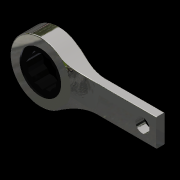
# Autodesk Inventor part: Ratchet
Saved by Autodesk Inventor 2014 SP1 (Build 180222100, 222)
## iProperties
Created: 2014-01-19
Part Number: Ratchet
Material: Generic
Document SubType Name: Modeling
Designer: Rauhul Varma
Mass: 5.86952 g
Surface Area: 33.2003 cm^2
Volume: 5.86952 cm^3
Density: 1 g/cm^3
Appearance: Steel - Polished
Author: Rauhul Varma
Autodesk Inventor part; units mm, degrees
ref_plane "YZ Plane" through (0, 0, 0) normal (1, 0, 0) x (0, 1, 0)
ref_plane "XZ Plane" through (0, 0, 0) normal (0, 1, 0) x (-1, 0, 0)
ref_plane "XY Plane" through (0, 0, 0) normal (0, 0, 1) x (1, 0, 0)
sketch "Sketch1" plane through (0, 0, 0) normal (0, 0, 1) x (1, 0, 0)
  arc A0 (12.3578, 6.35) -> (12.3578, -6.35) centre (0, 0) ccw
  line L0 (7.3323, 0) -> (3.6662, -6.35)
  line L1 (3.6662, -6.35) -> (-3.6662, -6.35)
  line L2 (-3.6662, -6.35) -> (-7.3323, 0)
  line L3 (-7.3323, 0) -> (-3.6662, 6.35)
  line L4 (-3.6662, 6.35) -> (3.6662, 6.35)
  line L5 (3.6662, 6.35) -> (7.3323, 0)
  line L6 (6.35, 3.6662) -> (6.35, -3.6662)
  line L7 (6.35, -3.6662) -> (0, -7.3323)
  line L8 (0, -7.3323) -> (-6.35, -3.6662)
  line L9 (-6.35, -3.6662) -> (-6.35, 3.6662)
  line L10 (-6.35, 3.6662) -> (0, 7.3323)
  line L11 (0, 7.3323) -> (6.35, 3.6662)
  line L12 (3.6662, 6.35) -> (12.3578, 6.35)
  line L13 (3.6662, -6.35) -> (12.3578, -6.35)
  line L14 (50.8, -6.35) -> (50.8, 6.35)
  line L15 (12.3578, 6.35) -> (50.8, 6.35)
  line L16 (12.3578, -6.35) -> (50.8, -6.35)
  arc A1 (12.3578, -6.35) -> (12.3578, 6.35) centre (0, 0) ccw
  dimension "d0" = 27.7876
  dimension "d1" = 12.7
  dimension "d2" = 12.7
  dimension "d14" = 50.8
  constraints: 34 end point, 4 parallel, 4 point on circle, 3 coincident, 2 centre point, 2 perpendicular, 2 vertical, 1 horizontal, 26 other
  measures "d0" diameter of A0
  measures "d1" distance between parallel lines of L1 L4
  measures "d2" distance between parallel lines of L8 L11
  measures "d14" distance from line of L14 A0.centre
extrude "Extrusion1" add sketch "Sketch1" along normal blind 4.3498 contours L12 L4 L11 L10 L3 L9 L2 L8 L1 L7 L13 A0 | A1 L13 L0 L7 L6 L5 L11 L12 | L5 L11 L4 | L1 L7 L0 | L11 L5 L6 L0 L7 L1 L8 L2 L9 L3 L10 L4 | L4 L10 L11 | L11 L6 L5 | L0 L6 L7 | L7 L8 L1 | L10 L3 L4 | L5 L0 L6 | L1 L2 L8 | L3 L9 L10 | L8 L9 L2 | L9 L2 L3
extrude "Extrusion2" add sketch "Sketch1" along normal blind 1.9685 contours A1 L13 L0 L7 L6 L5 L11 L12 | L15 L14 L16 A1 | L11 L6 L5 | L0 L6 L7
fillet "Fillet1" radius 25.4 3 edges at (12.3578, 6.35, 0.9842) (12.3578, -6.35, 0.9842) (13.8938, 0, 1.9685)
fillet "Fillet2" radius 0.3969 7 edges at (23.4746, 6.35, 1.9704) (15.2626, 7.6058, 3.1255) (37.2994, 6.35, 1.9685) (-13.8938, 0, 4.3498) (23.4746, -6.35, 1.9704) (37.2994, -6.35, 1.9685) (15.2626, -7.6058, 3.1255)
extrude "Extrusion3" cut sketch "Sketch1" along normal through all contours L5 L11 L4 | L1 L7 L0 | L11 L5 L6 L0 L7 L1 L8 L2 L9 L3 L10 L4 | L4 L10 L11 | L11 L6 L5 | L0 L6 L7 | L7 L8 L1 | L10 L3 L4 | L5 L0 L6 | L1 L2 L8 | L3 L9 L10 | L8 L9 L2 | L9 L2 L3
sketch "Sketch2" plane through (0, 0, 4.3498) normal (0, 0, 1) x (1, 0, 0)
  arc A0 (10.1891, -9.4457) -> (10.1891, 9.4457) centre (0, 0) ccw projected
  line L0 (6.35, 3.6662) -> (6.35, -3.6662) projected
  line L1 (6.35, -3.6662) -> (0, -7.3323) projected
  line L2 (4.6485, -4.6485) -> (3.6662, -6.35) projected
  line L3 (3.6662, -6.35) -> (1.7015, -6.35) projected
  line L4 (6.35, -3.6662) -> (0, -7.3323) projected
  line L5 (0, -7.3323) -> (-6.35, -3.6662) projected
  line L6 (-1.7015, -6.35) -> (-3.6662, -6.35) projected
  line L7 (-3.6662, -6.35) -> (-4.6485, -4.6485) projected
  line L8 (0, -7.3323) -> (-6.35, -3.6662) projected
  line L9 (-6.35, -3.6662) -> (-6.35, 3.6662) projected
  line L10 (-6.35, -1.7015) -> (-7.3323, 0) projected
  line L11 (-7.3323, 0) -> (-6.35, 1.7015) projected
  line L12 (-6.35, -3.6662) -> (-6.35, 3.6662) projected
  line L13 (-6.35, 3.6662) -> (0, 7.3323) projected
  line L14 (-4.6485, 4.6485) -> (-3.6662, 6.35) projected
  line L15 (-3.6662, 6.35) -> (-1.7015, 6.35) projected
  line L16 (-6.35, 3.6662) -> (0, 7.3323) projected
  line L17 (0, 7.3323) -> (6.35, 3.6662) projected
  line L18 (1.7015, 6.35) -> (3.6662, 6.35) projected
  line L19 (3.6662, 6.35) -> (4.6485, 4.6485) projected
  line L20 (0, 7.3323) -> (6.35, 3.6662) projected
  line L21 (6.35, 3.6662) -> (6.35, -3.6662) projected
  line L22 (6.35, 1.7015) -> (7.3323, 0) projected
  line L23 (7.3323, 0) -> (6.35, -1.7015) projected
  circle A1 centre (0, 0) radius 9.525
  dimension "d11" = 19.05
  constraints: 1 centre point, 1 coincident
  measures "d11" diameter of A1
extrude "Extrusion4" cut sketch "Sketch2" against normal blind 0.7937
sketch "Sketch3" plane through (0, 0, 0) normal (0, 0, -1) x (-1, 0, 0)
  line L0 (-50.8, -6.35) -> (-50.8, 6.35) projected
  line L1 (-50.8, 0) -> (-44.45, 0) construction
  dimension "d15" = 6.35
  constraints: 2 end point, 1 horizontal, 1 midpoint
  measures "d15" distance from line of L0 L1.end
hole "Hole1" at (44.45, 0, 0) direction (0, 0, 1) diameter 6.5278 end through all clearance for "Socket Head Cap Screw" size "1/4" standard "Ansi Unified Screw Threads"
mirror "Mirror1" about plane through (8.399, 0, 0) normal (0, 0, -1)
body "Solid1"
